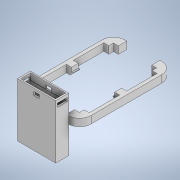
# Autodesk Inventor part: Extension
Saved by Autodesk Inventor 2020 (Build 240168000, 168)
## iProperties
Created: 2021-10-27
Part Number: Extension
Material: Типовые
Document SubType Name: Modeling
Designer: User
Density: 1 g/cm^3
Appearance: По умолчанию
Author: User
Autodesk Inventor part; units mm, degrees
ref_plane "YZ Plane" through (0, 0, 0) normal (1, 0, 0) x (0, 1, 0)
ref_plane "XZ Plane" through (0, 0, 0) normal (0, 1, 0) x (-1, 0, 0)
ref_plane "XY Plane" through (0, 0, 0) normal (0, 0, 1) x (1, 0, 0)
sketch "Эскиз1" plane through (0, 0, 0) normal (0, 1, 0) x (-1, 0, 0)
  line L0 (0, 0) -> (9.1667, 0)
  line L1 (0, 0) -> (0, -12.5)
  line L2 (-11.2667, 28.6) -> (11.2667, 28.6)
  line L3 (18.2667, 21.6) -> (18.2667, -21.6)
  line L4 (-18.2667, -21.6) -> (-18.2667, 21.6)
  line L5 (13.1667, -2.1) -> (16.2667, -2.1)
  line L6 (16.2667, -2.1) -> (16.2667, -20.7)
  line L7 (16.2667, -20.7) -> (13.1667, -20.7)
  line L8 (13.1667, 2.1) -> (16.2667, 2.1)
  line L9 (16.2667, 2.1) -> (16.2667, 20.7)
  line L10 (16.2667, 20.7) -> (13.1667, 20.7)
  line L11 (-16.2667, 2.1) -> (-16.2667, 20.7)
  line L12 (-16.2667, 20.7) -> (-13.1667, 20.7)
  line L13 (-13.1667, 2.1) -> (-16.2667, 2.1)
  line L14 (-13.1667, -2.1) -> (-16.2667, -2.1)
  line L15 (-16.2667, -2.1) -> (-16.2667, -20.7)
  line L16 (-16.2667, -20.7) -> (-13.1667, -20.7)
  line L17 (10.1667, -23.5) -> (10.1667, -26.6)
  line L18 (-10.1667, -26.6) -> (-10.1667, -23.5)
  line L19 (10.1667, 23.5) -> (10.1667, 26.6)
  line L20 (10.1667, 26.6) -> (-10.1667, 26.6)
  line L21 (-10.1667, 26.6) -> (-10.1667, 23.5)
  arc A0 (18.2667, 21.6) -> (11.2667, 28.6) centre (11.2667, 21.6) ccw
  arc A1 (-11.2667, 28.6) -> (-18.2667, 21.6) centre (-11.2667, 21.6) ccw
  arc A2 (-18.2667, -21.6) -> (-11.2667, -28.6) centre (-11.2667, -21.6) ccw
  arc A3 (11.2667, -28.6) -> (18.2667, -21.6) centre (11.2667, -21.6) ccw
  line L22 (-10.1667, -26.6) -> (-10.1667, -28.6)
  line L23 (-10.1667, -28.6) -> (-11.2667, -28.6)
  line L24 (10.1667, -26.6) -> (10.1667, -28.6)
  line L25 (10.1667, -28.6) -> (11.2667, -28.6)
  line L26 (-10.1667, 23.5) -> (-13.1667, 23.5)
  line L27 (-13.1667, 23.5) -> (-13.1667, 20.7)
  line L28 (10.1667, 23.5) -> (13.1667, 23.5)
  line L29 (13.1667, 23.5) -> (13.1667, 20.7)
  line L30 (-10.1667, -23.5) -> (-13.1667, -23.5)
  line L31 (-13.1667, -23.5) -> (-13.1667, -20.7)
  line L32 (10.1667, -23.5) -> (13.1667, -23.5)
  line L33 (13.1667, -23.5) -> (13.1667, -20.7)
  line L34 (13.1667, 2.1) -> (13.1667, -2.1)
  line L35 (-13.1667, 2.1) -> (-13.1667, -2.1)
  constraints: 72 end point, 20 symmetric about line, 8 point on circle, 6 tangent, 4 centre point, 4 horizontal, 3 equal radius, 2 perpendicular, 2 vertical, 1 parallel
extrude "Выдавливание1" add sketch "Эскиз1" along normal blind 4.5
sketch "Эскиз2" plane through (-13.1667, 0, 2.1) normal (1, 0, 0) x (0, 0, -1)
  line L0 (-18.6, 0) -> (0, 0) projected
  line L1 (4.2, 0) -> (4.2, 4.5) projected
  line L2 (0, 0) -> (4.2, 0)
  line L3 (4.2, 0) -> (4.2, 2)
  line L4 (4.2, 2) -> (0, 2)
  line L5 (0, 2) -> (0, 0)
  point P0 (2.1, 0)
  dimension "d19" = 2
  constraints: 8 end point, 2 parallel, 1 horizontal, 1 perpendicular, 1 point on line
  measures "d19" distance between parallel lines of L2 L4
extrude "Выдавливание2" add sketch "Эскиз2" along normal blind 1
chamfer "Фаска1" distance 1.8 angle 45 1 edges at (-12.1667, 0, 0)
mirror "Зеркальное отражение1" about plane through (0, 0, 0) normal (1, 0, 0) of "Выдавливание2", "Фаска1"
sketch "Эскиз3" plane through (-11.2667, 0, 28.6) normal (0, 0, 1) x (1, 0, 0)
  line L0 (1.1, 4.5) -> (-1.9, 4.5) projected
  line L1 (21.4333, 0) -> (24.4333, 0) projected
  line L2 (-0.4, 4.5) -> (22.9333, 4.5)
  line L3 (22.9333, 4.5) -> (22.9333, 0)
  line L4 (22.9333, 0) -> (-0.4, 0)
  line L5 (-0.4, 0) -> (-0.4, 4.5)
  point P0 (11.2667, 0)
  constraints: 8 end point, 2 midpoint, 2 parallel, 1 horizontal, 1 perpendicular
extrude "Выдавливание3" add sketch "Эскиз3" along normal blind 7.9
sketch "Эскиз4" plane through (0, 4.5, 0) normal (0, 1, 0) x (1, 0, 0)
  line L0 (-11.2667, -28.6) -> (-11.6667, -28.6) projected
  line L1 (11.6667, -36.5) -> (-11.6667, -36.5) projected
  line L2 (-11.6667, -28.6) -> (11.6667, -28.6)
  line L3 (11.6667, -28.6) -> (11.6667, -36.5)
  line L4 (11.6667, -36.5) -> (-11.6667, -36.5)
  line L5 (-11.6667, -36.5) -> (-11.6667, -28.6)
  point P0 (0, 0)
  constraints: 8 end point, 2 parallel, 1 horizontal, 1 perpendicular
extrude "Выдавливание4" add sketch "Эскиз4" against normal blind 21
sketch "Эскиз5" plane through (0, 4.5, 0) normal (0, 1, 0) x (1, 0, 0)
  line L0 (-10.6667, -35.5) -> (10.6667, -35.5)
  line L1 (10.6667, -35.5) -> (10.6667, -29.6)
  line L2 (10.6667, -29.6) -> (-10.6667, -29.6)
  line L3 (-10.6667, -29.6) -> (-10.6667, -35.5)
  line L4 (-11.6667, -28.6) -> (-11.6667, -36.5) projected
  line L5 (11.6667, -28.6) -> (11.6667, -36.5) projected
  line L6 (11.6667, -36.5) -> (-11.6667, -36.5) projected
  line L7 (11.2667, -28.6) -> (-11.2667, -28.6) projected
  point P0 (0, 0)
  dimension "d29" = 1
  dimension "d30" = 1
  dimension "d31" = 1
  dimension "d32" = 1
  constraints: 8 end point, 2 parallel, 1 horizontal, 1 perpendicular
  measures "d29" distance between parallel lines of L3 L4
  measures "d30" distance between parallel lines of L5 L1
  measures "d31" distance between parallel lines of L6 L0
  measures "d32" distance between parallel lines of L7 L2
extrude "Выдавливание5" cut sketch "Эскиз5" against normal blind 20
sketch "Эскиз6" plane through (0, 4.5, 0) normal (0, 1, 0) x (1, 0, 0)
  line L0 (-11.6667, -28.6) -> (-11.6667, -36.5) projected
  line L1 (11.6667, -28.6) -> (11.2667, -28.6) projected
  line L2 (-11.6667, -28.6) -> (11.6667, -28.6)
  line L3 (-11.6667, -28.6) -> (-11.6667, -36.5)
  line L4 (11.6667, -36.5) -> (-11.6667, -36.5) projected
  line L5 (11.6667, -28.6) -> (11.6667, -36.5) projected
  line L6 (11.6667, -36.5) -> (11.6667, -28.6)
  line L7 (11.6667, -36.5) -> (-11.6667, -36.5)
  line L8 (-10.6667, -29.6) -> (10.6667, -29.6) projected
  line L9 (10.6667, -29.6) -> (10.6667, -35.5) projected
  line L10 (-10.6667, -29.6) -> (10.6667, -29.6)
  line L11 (10.6667, -29.6) -> (10.6667, -35.5)
  line L12 (10.6667, -35.5) -> (-10.6667, -35.5)
  line L13 (-10.6667, -35.5) -> (-10.6667, -29.6)
  point P0 (0, 0)
  constraints: 16 end point, 4 equal length, 2 horizontal, 2 perpendicular
extrude "Выдавливание6" add sketch "Эскиз6" along normal blind 8
sketch "Эскиз7" plane through (0, 12.5, 0) normal (0, 1, 0) x (1, 0, 0)
  line L0 (-11.6667, -36.5) -> (-11.6667, -28.6) projected
  line L1 (11.6667, -36.5) -> (-11.6667, -36.5) projected
  line L2 (-11.6667, -28.6) -> (11.6667, -28.6)
  line L3 (11.6667, -28.6) -> (11.6667, -36.5)
  line L4 (11.6667, -36.5) -> (-11.6667, -36.5)
  line L5 (-11.6667, -36.5) -> (-11.6667, -28.6)
  line L6 (10.6667, -29.6) -> (10.6667, -35.5)
  line L7 (-10.6667, -35.5) -> (-10.6667, -29.6)
  line L8 (11.2667, -28.6) -> (-11.2667, -28.6) projected
  line L9 (-1.6667, -28.6) -> (1.6667, -28.6)
  line L10 (-10.6667, -29.6) -> (-11.6667, -29.6)
  line L11 (-10.6667, -35.5) -> (-11.6667, -35.5)
  line L12 (10.6667, -35.5) -> (11.6667, -35.5)
  line L13 (10.6667, -29.6) -> (11.6667, -29.6)
  line L14 (1.6667, -36.5) -> (-1.6667, -36.5)
  line L15 (-10.6667, -35.5) -> (-10.6667, -29.6) projected
  line L16 (-10.6667, -29.6) -> (-10.6667, -29.4)
  line L17 (-10.6667, -29.4) -> (10.6667, -29.4)
  line L18 (10.6667, -29.4) -> (10.6667, -29.6)
  line L19 (-10.6667, -35.5) -> (-10.6667, -35.7)
  line L20 (-10.6667, -35.7) -> (10.6667, -35.7)
  line L21 (10.6667, -35.7) -> (10.6667, -35.5)
  line L22 (-1.6667, -28.6) -> (1.6667, -28.6)
  line L23 (1.6667, -28.6) -> (1.6667, -29.4)
  line L24 (1.6667, -29.4) -> (-1.6667, -29.4)
  line L25 (-1.6667, -29.4) -> (-1.6667, -28.6)
  line L26 (-1.6667, -35.7) -> (1.6667, -35.7)
  line L27 (1.6667, -35.7) -> (1.6667, -36.5)
  line L28 (1.6667, -36.5) -> (-1.6667, -36.5)
  line L29 (-1.6667, -36.5) -> (-1.6667, -35.7)
  point P0 (0, 0)
  dimension "d42" = 0.8
  dimension "d43" = 0.8
  dimension "d44" = 10
  dimension "d45" = 10
  dimension "d46" = 10
  dimension "d47" = 10
  constraints: 52 end point, 12 point on line, 8 parallel, 8 perpendicular, 4 horizontal, 1 vertical
  measures "d42" distance between parallel lines of L17 L8
  measures "d43" distance between parallel lines of L1 L20
  measures "d44" distance between parallel lines of L3 L23
  measures "d45" distance between parallel lines of L0 L25
  measures "d46" distance between parallel lines of L0 L29
  measures "d47" distance between parallel lines of L3 L27
extrude "Выдавливание7" add sketch "Эскиз7" along normal blind 4 contours L0 L11 L19 L20 L29 L1 | L0 L2 L25 L17 L16 L10 | L27 L20 L21 L12 L3 L1 | L13 L18 L17 L23 L2 L3
sketch "Эскиз8" plane through (0, 16.5, 0) normal (0, 1, 0) x (1, 0, 0)
  line L0 (-11.6667, -28.6) -> (-11.6667, -29.6) projected
  line L1 (11.6667, -36.5) -> (-11.6667, -36.5) projected
  line L2 (-11.6667, -28.6) -> (11.6667, -28.6)
  line L3 (11.6667, -28.6) -> (11.6667, -36.5)
  line L4 (11.6667, -36.5) -> (-11.6667, -36.5)
  line L5 (-11.6667, -36.5) -> (-11.6667, -28.6)
  line L6 (-10.6667, -29.4) -> (-1.6667, -29.4) projected
  line L7 (10.6667, -35.7) -> (1.6667, -35.7) projected
  line L8 (-10.6667, -29.4) -> (10.6667, -29.4)
  line L9 (10.6667, -29.4) -> (10.6667, -35.7)
  line L10 (10.6667, -35.7) -> (-10.6667, -35.7)
  line L11 (-10.6667, -35.7) -> (-10.6667, -29.4)
  point P0 (0, 0)
  constraints: 16 end point, 4 parallel, 2 horizontal, 2 perpendicular
extrude "Выдавливание8" add sketch "Эскиз8" against normal blind 1.8
